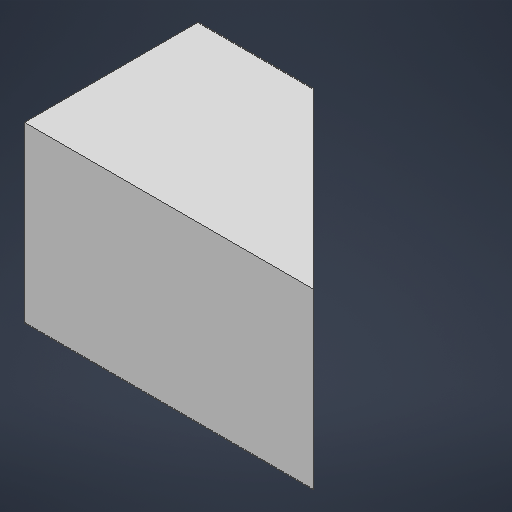
# Autodesk Inventor part: cajon_1_proyecto_diseno
Saved by Autodesk Inventor 2027 (Build 310192000, 192)
## iProperties
Created: 2026-04-28
Part Number: cajon_1_proyecto_diseno
Material: Genérico
Document SubType Name: Modeling
Designer: agusb
Density: 1 g/cm^3
Appearance: Valor por defecto
Author: agusb
Autodesk Inventor part; units mm, degrees
ref_plane "YZ Plane" through (0, 0, 0) normal (1, 0, 0) x (0, 1, 0)
ref_plane "XZ Plane" through (0, 0, 0) normal (0, 1, 0) x (-1, 0, 0)
ref_plane "XY Plane" through (0, 0, 0) normal (0, 0, 1) x (1, 0, 0)
sketch "Boceto1" plane through (0, 0, 0) normal (0, 1, 0) x (-1, 0, 0)
  line L0 (0, 0) -> (0, -350)
  line L1 (0, -350) -> (-350, 0)
  line L2 (-350, 0) -> (0, 0)
  dimension "d0" = 350
  dimension "d1" = 45
  constraints: 6 end point, 1 perpendicular, 1 vertical
  measures "d0" distance of L0.start L0.end
  measures "d1" angle of L0 L1
extrude "Extrusión1" add sketch "Boceto1" along normal blind 1
sketch "Boceto2" plane through (0, 1, 0) normal (0, 1, 0) x (1, 0, 0)
  line L0 (350, 0) -> (0, 350) projected
  line L1 (350, 0) -> (349, 0)
  line L2 (0, 0) -> (350, 0) projected
  line L3 (0, 350) -> (0, 349)
  line L4 (0, 350) -> (0, 0) projected
  line L5 (0, 0) -> (0, 1)
  line L6 (0, 0) -> (1, 0)
  line L7 (349, 0) -> (0, 349)
  line L8 (1, 0) -> (1, 348)
  line L9 (0, 1) -> (348, 1)
  dimension "d4" = 1
  dimension "d5" = 1
  dimension "d6" = 1
  dimension "d7" = 1
  constraints: 14 end point, 6 point on line, 1 parallel, 1 perpendicular
  measures "d4" distance of L0.start L1.end
  measures "d5" distance of L0.end L3.end
  measures "d6" distance of L2.start L5.end
  measures "d7" distance of L2.start L6.end
extrude "Extrusión2" add sketch "Boceto2" along normal blind 348 contours L1 L7 L3 L0 | L2 L8 L9 L7 | L2 L4 L9 L8
sketch "Boceto3" plane through (0, 349, 0) normal (0, 1, 0) x (1, 0, 0)
  line L0 (0, 350) -> (0, 0) projected
  line L1 (0, 0) -> (0, 350)
  line L2 (0, 0) -> (350, 0) projected
  line L3 (0, 350) -> (350, 0)
  line L4 (350, 0) -> (0, 0)
  constraints: 6 end point, 2 collinear
extrude "Extrusión3" add sketch "Boceto3" along normal blind 1
sketch "Boceto4" plane through (0, 0, -350) normal (-1, 0, 0) x (0, 0, 1)
  line L0 (349, 1) -> (349, 349) projected
  line L1 (349, 1) -> (349, 349)
  line L2 (1, 1) -> (1, 349) projected
  line L3 (349, 349) -> (1, 349)
  line L4 (1, 349) -> (1, 1)
  line L5 (1, 1) -> (349, 1)
  line L6 (0, 0) -> (0, 350) projected
  line L7 (0, 350) -> (350, 350)
  line L8 (350, 0) -> (350, 350) projected
  line L9 (350, 350) -> (350, 0)
  line L10 (350, 0) -> (0, 0) projected
  line L11 (350, 0) -> (0, 0)
  line L12 (0, 0) -> (0, 350)
  constraints: 16 end point, 4 perpendicular, 2 collinear, 1 horizontal, 1 parallel
extrude "Extrusión4" add sketch "Boceto4" along normal blind 233.1
